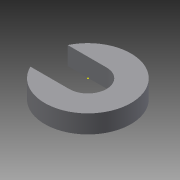
# Autodesk Inventor part: reinforce
Saved by Autodesk Inventor 2015 SP2 (Build 190223200, 223)
## iProperties
Created: 2016-02-23
Part Number: reinforce
Material: Generic
Document SubType Name: Modeling
Designer: Brandon
Density: 1 g/cm^3
Appearance: Default
Author: Brandon
Autodesk Inventor part; units mm, degrees
ref_plane "YZ Plane" through (0, 0, 0) normal (1, 0, 0) x (0, 1, 0)
ref_plane "XZ Plane" through (0, 0, 0) normal (0, 1, 0) x (-1, 0, 0)
ref_plane "XY Plane" through (0, 0, 0) normal (0, 0, 1) x (1, 0, 0)
sketch "Sketch1" plane through (0, 0, 0) normal (0, 0, 1) x (1, 0, 0)
  arc A0 (-13.5185, -6.5) -> (-13.5185, 6.5) centre (0, 0) ccw
  arc A1 (0, -6.5) -> (0, 6.5) centre (0, 0) ccw
  line L0 (0, -6.5) -> (-13.5185, -6.5)
  line L1 (0, 6.5) -> (-13.5185, 6.5)
  line L2 (-13.5185, 6.5) -> (-12.5, 6.5)
  dimension "d0" = 30
  dimension "d1" = 13
  constraints: 6 end point, 4 point on circle, 2 centre point, 2 coincident, 2 horizontal, 2 tangent, 1 point on line
  measures "d0" diameter of A0
  measures "d1" diameter of A1
extrude "Extrusion1" add sketch "Sketch1" along normal blind 6.35
sketch "Sketch2" plane through (0, 0, 0) normal (0, 0, -1) x (-1, 0, 0)
  point P0 (0, 0)
sketch "Sketch3" plane through (0, 0, 6.35) normal (0, 0, 1) x (1, 0, 0)
  point P0 (0, 0)
body "Solid1"
